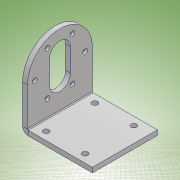
# Autodesk Inventor part: 零件41
Saved by Autodesk Inventor 2017 (Build 210142000, 142)
## iProperties
Part Number: 零件41
Material: 常规
Document SubType Name: 钣金
Designer: ZYB
Density: 1 g/cm^3
Sheet Metal Rule: 默认_mm
Appearance: 默认
Mass: 8.55024 g
Surface Area: 69.3805 cm^2
Volume: 8.55024 cm^3
Author: ZYB
Autodesk Inventor part; units mm, degrees
ref_plane "YZ Plane" through (0, 0, 0) normal (1, 0, 0) x (0, 1, 0)
ref_plane "XZ Plane" through (0, 0, 0) normal (0, 1, 0) x (-1, 0, 0)
ref_plane "XY Plane" through (0, 0, 0) normal (0, 0, 1) x (1, 0, 0)
sketch "草图1" plane through (0, 0, 0) normal (0, 0, 1) x (1, 0, 0)
  line L0 (21.5, -20) -> (-21.5, -20)
  line L1 (-21.5, -20) -> (-21.5, 20)
  line L2 (-21.5, 20) -> (21.5, 20)
  line L3 (21.5, 20) -> (21.5, -20)
  line L4 (21.5, -20) -> (-21.5, 20) construction
  line L5 (-21.5, -20) -> (21.5, 20) construction
  line L6 (12, -15) -> (-12, -15) construction
  line L7 (-12, -15) -> (-12, 15) construction
  line L8 (-12, 15) -> (12, 15) construction
  line L9 (12, 15) -> (12, -15) construction
  line L10 (12, -15) -> (-12, 15) construction
  line L11 (-12, -15) -> (12, 15) construction
  circle A0 centre (-12, 15) radius 1.75
  circle A1 centre (12, 15) radius 1.75
  circle A2 centre (-12, -15) radius 1.75
  circle A3 centre (12, -15) radius 1.75
  point P0 (0, 0)
  dimension "d0" = 43
  dimension "d1" = 40
  dimension "d2" = 3.5
  dimension "d3" = 24
  dimension "d4" = 30
  measures "d0" distance of L1.end L2.end
  measures "d1" distance of L2.end L0.start
  measures "d2" diameter of A0
  measures "d3" distance of L7.end L8.end
  measures "d4" distance of L6.end L7.end
extrude "平板1" add sketch "草图1" along normal blind 3
sketch "草图2" plane through (-18.5, -20, 0) normal (-1, 0, 0) x (0, -1, 0)
  line L0 (-40, 0) -> (0, 0)
  line L1 (0, 0) -> (0, 47)
  line L2 (0, 47) -> (-40, 47)
  line L3 (-40, 47) -> (-40, 0)
  constraints: 6 end point, 1 horizontal, 1 perpendicular, 1 vertical
edge flange "凸缘1" height 47 angle 90 thickness 3 bend radius 0.5 thickness toward (-1, 0, 0) relief straight relief width 3 relief depth 1.5 edges at (-21.5, 0, 3) wall of the first edge with corners at (-18.5, 20, 0) (-18.5, -20, 0) (-18.5, -20, 47) (-18.5, 20, 47)
bend "折弯1"
corner "拐角1"
sketch "草图3" plane through (-21.5, -20, 47) normal (-1, 0, 0) x (0, 0, 1)
  line L0 (-27, 20) -> (-13, 20) construction
  line L1 (-27, 13.5) -> (-13, 13.5)
  line L2 (-13, 26.5) -> (-27, 26.5)
  arc A0 (-27, 26.5) -> (-27, 13.5) centre (-27, 20) ccw
  arc A1 (-13, 13.5) -> (-13, 26.5) centre (-13, 20) ccw
  line L3 (-47, 0) -> (-47, 40) projected
  point P0 (-47, 20)
  point P1 (-20, 20)
  point P2 (-47, 20)
  dimension "d16" = 27
  dimension "d17" = 27
  dimension "d18" = 13
  constraints: 8 end point, 4 point on circle, 4 tangent, 2 centre point, 2 midpoint, 1 horizontal, 1 parallel, 1 point on line
  measures "d16" distance from line of L3 point (-20, 20)
  measures "d18" distance between parallel lines of L1 L2
extrude "拉伸1" cut sketch "草图3" against normal blind 10
fillet "圆角1" radius 20 2 edges at (-20, -20, 47) (-20, 20, 47)
sketch "草图4" plane through (-21.5, -20, 3.5) normal (-1, 0, 0) x (0, 0, 1)
  circle A0 centre (23.5, 35.5) radius 1.5
  arc A1 (23.5, 0) -> (23.5, 40) centre (23.5, 20) ccw projected
  line L0 (0, 40) -> (23.5, 40) projected
  line L1 (0, 40) -> (0, 0) projected
  line L2 (23.5, 0) -> (0, 0) projected
  arc A2 (30.5, 13.5) -> (30.5, 26.5) centre (30.5, 20) ccw projected
  line L3 (30.5, 13.5) -> (16.5, 13.5) projected
  arc A3 (16.5, 26.5) -> (16.5, 13.5) centre (16.5, 20) ccw projected
  line L4 (16.5, 26.5) -> (30.5, 26.5) projected
  point P0 (-3.5, 20)
  dimension "d22" = 15.5
  dimension "d23" = 3
  constraints: 1 centre point, 1 vertical alignment
  measures "d22" distance of A0.centre A1.centre
  measures "d23" diameter of A0
extrude "拉伸2" cut sketch "草图4" against normal blind 10 contours A0
chamfer "倒角1" distance 1.5 angle 45 1 edges at (-21.5, 15.5, 25.5)
pattern_circular "环形阵列1" count 6 over 360 about axis through (-18.5, 0, 27) along (-1, 0, 0) of "拉伸2", "倒角1"
equation "\"d6\" = 折弯释压宽度"
equation "\"d7\" = 折弯释压深度"
equation "\"d8\" = 最小余量"
equation "\"d9\" = 折弯半径"
equation "\"d13\" = 拐角释压尺寸"
equation "\"d14\" = 间隙大小"
equation "\"d15\" = Jacobi半径尺寸"
equation "\"折弯半径\" = 厚度"
equation "\"折弯释压宽度\" = 厚度"
equation "\"折弯释压深度\" = 0.5 * 厚度"
equation "\"拐角释压尺寸\" = 4 * 厚度"
equation "\"最小余量\" = 2 * 厚度"
equation "\"过渡半径\" = 折弯半径"
equation "\"Jacobi半径尺寸\" = 折弯半径"
equation "\"间隙大小\" = 厚度"
equation "\"d5\" = 折弯半径"
equation "\"厚度\" = 3"
